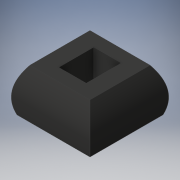
# Autodesk Inventor part: keyswitch-base_cherrymx
Saved by Autodesk Inventor 2016 (Build 200138000, 138)
## iProperties
Created: 2016-12-08
Part Number: keyswitch-base_cherrymx
Material: Generic
Document SubType Name: Modeling
Designer: Cemra JC
Density: 1 g/cm^3
Appearance: Default
Author: Cemra JC
Autodesk Inventor part; units mm, degrees
ref_plane "YZ Plane" through (0, 0, 0) normal (1, 0, 0) x (0, 1, 0)
ref_plane "XZ Plane" through (0, 0, 0) normal (0, 1, 0) x (-1, 0, 0)
sketch "Base Loop" plane through (0, 0, 0) normal (0, 1, 0) x (-1, 0, 0)
  line L0 (-7.3, 7.3) -> (7.3, 7.3)
  line L1 (7.3, 7.3) -> (7.3, -7.3)
  line L2 (7.3, -7.3) -> (-7.3, -7.3)
  line L3 (-7.3, -7.3) -> (-7.3, 7.3)
  line L4 (-7.3, 7.3) -> (7.3, -7.3) construction
  line L5 (7.3, 7.3) -> (-7.3, -7.3) construction
  point P0 (0, 0)
  point P1 (0, 0)
  point P2 (0, 0)
  dimension "d0" = 14.6
  dimension "d1" = 14.6
  constraints: 12 end point, 3 midpoint, 2 parallel, 1 coincident, 1 horizontal, 1 perpendicular
  measures "d0" distance of L1.end L2.end
  measures "d1" distance of L0.end L1.end
ref_plane "Mid Plane" through (-7.3, 2, -7.3) normal (0, 1, 0) x (1, 0, 0)
ref_plane "Base Plane" through (-7.3, 0, -7.3) normal (0, 1, 0) x (1, 0, 0)
sketch "Mid Loop" plane through (-7.3, 2, -7.3) normal (0, 1, 0) x (1, 0, 0)
  line L0 (15.1, -15.1) -> (-0.5, -15.1)
  line L1 (-0.5, -15.1) -> (-0.5, 0.5)
  line L2 (-0.5, 0.5) -> (15.1, 0.5)
  line L3 (15.1, 0.5) -> (15.1, -15.1)
  line L4 (15.1, -15.1) -> (-0.5, 0.5) construction
  line L5 (-0.5, -15.1) -> (15.1, 0.5) construction
  point P0 (7.3, -7.3)
  dimension "d3" = 15.6
  dimension "d4" = 15.6
  constraints: 12 end point, 2 midpoint, 2 parallel, 1 horizontal, 1 perpendicular
  measures "d3" distance of L0.end L1.end
  measures "d4" distance of L1.end L2.end
ref_plane "Top Plane" through (-7.3, 8.6, -7.3) normal (0, 1, 0) x (1, 0, 0)
sketch "Top Loop" plane through (-7.3, 8.6, -7.3) normal (0, 1, 0) x (1, 0, 0)
  line L0 (13.3, -13.3) -> (1.3, -13.3)
  line L1 (1.3, -13.3) -> (1.3, -1.3)
  line L2 (1.3, -1.3) -> (13.3, -1.3)
  line L3 (13.3, -1.3) -> (13.3, -13.3)
  line L4 (13.3, -13.3) -> (1.3, -1.3) construction
  line L5 (1.3, -13.3) -> (13.3, -1.3) construction
  point P0 (7.3, -7.3)
  dimension "d6" = 12
  dimension "d7" = 12
  constraints: 12 end point, 2 midpoint, 2 parallel, 1 horizontal, 1 perpendicular
  measures "d6" distance of L1.end L2.end
  measures "d7" distance of L0.end L1.end
loft "Keyswitch Body" add profiles "Base Loop", "Mid Loop", "Top Loop"
sketch "Cut in profile" plane through (-6, 8.6, 6) normal (0, 1, 0) x (1, 0, 0)
  line L0 (8.75, 2.5) -> (3.25, 2.5)
  line L1 (3.25, 2.5) -> (3.25, 9.5)
  line L2 (3.25, 9.5) -> (8.75, 9.5)
  line L3 (8.75, 9.5) -> (8.75, 2.5)
  line L4 (8.75, 2.5) -> (3.25, 9.5) construction
  line L5 (3.25, 2.5) -> (8.75, 9.5) construction
  point P0 (6, 6)
  dimension "d17" = 7
  dimension "d18" = 5.5
  constraints: 12 end point, 2 midpoint, 2 parallel, 1 horizontal, 1 perpendicular
  measures "d17" distance of L0.end L1.end
  measures "d18" distance of L0.start L0.end
extrude "Pole Cut in" cut sketch "Cut in profile" against normal blind 6.6
equation "\"d1\" = d0"
equation "\"d3\" = s_bwidth"
equation "\"d4\" = d3"
equation "\"d17\" = s_polebl"
equation "\"d18\" = s_polebw"
equation "\"k_width\" = 18.1"
equation "\"k_height\" = 18"
equation "\"k_taper1\" = 1.5"
equation "\"k_taper2\" = 0.5"
equation "\"k_radius\" = 6"
equation "\"k_wthick\" = 1.5"
equation "\"k_ribthick\" = 1.5"
equation "\"k_ribheight\" = 5"
equation "\"k_poleoff\" = 2.2625"
equation "\"k_poledia\" = 5.54"
equation "\"k_cmxw\" = 1.6"
equation "\"k_cmxl\" = 4.35"
equation "\"s_bwidth\" = 15.6"
equation "\"s_poleh\" = 3.6"
equation "\"s_polebw\" = 5.5"
equation "\"s_polebl\" = 7"
equation "\"b_rshift\" = 49.775"
equation "\"b_ctrl\" = 22.625"
equation "\"b_space\" = 117.65"
equation "\"b_height\" = 77.4"
equation "\"b_width\" = 286.5"
equation "\"b_lshift\" = 40.725"
equation "\"b_tab\" = 27.15"
equation "\"b_pad\" = 1"
equation "\"b_caps\" = 31.675"
equation "\"k_staper\" = 1"
equation "\"k_ltaper\" = 1.5"
equation "\"k_lradius\" = 6"
equation "\"k_sradius\" = 4"
equation "\"k_height_t\" = 16"
equation "\"k_taper_wide\" = 1.5"
equation "\"k_taper_thin\" = 0.5"
equation "\"k_height_low\" = 16"
body "Solid1"
